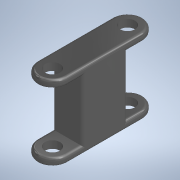
# Autodesk Inventor part: Link2
Saved by Autodesk Inventor 2022 (Build 260153000, 153)
## iProperties
Part Number: Link2
Material: Generic
Document SubType Name: Modeling
Designer: suhas
Appearance: Default
Author: suhas
Autodesk Inventor part; units mm, degrees
ref_plane "YZ Plane" through (0, 0, 0) normal (1, 0, 0) x (0, 1, 0)
ref_plane "XZ Plane" through (0, 0, 0) normal (0, 1, 0) x (-1, 0, 0)
ref_plane "XY Plane" through (0, 0, 0) normal (0, 0, 1) x (1, 0, 0)
sketch "Sketch1" plane through (0, 0, 0) normal (0, 1, 0) x (-1, 0, 0)
  line L0 (10, -25) -> (10, 25)
  line L1 (-10, 25) -> (-10, -25)
  arc A0 (10, 25) -> (-10, 25) centre (0, 25) ccw
  arc A1 (-10, -25) -> (10, -25) centre (0, -25) ccw
  circle A2 centre (0, 25) radius 5
  circle A3 centre (0, -25) radius 5
  point P0 (0, 0)
  constraints: 4 centre point, 4 end point, 4 point on circle, 2 coincident, 1 parallel, 1 tangent
extrude "Extrusion1" add sketch "Sketch1" along normal blind 50
sketch "Sketch2" plane through (-10, 0, -25) normal (-1, 0, 0) x (0, 0, 1)
  line L0 (-10, 0) -> (-10, 50) projected
  line L1 (10, 5) -> (-10, 5)
  line L2 (-10, 5) -> (-10, 45)
  line L3 (-10, 45) -> (10, 45)
  line L4 (10, 45) -> (10, 5)
  line L5 (0, 0) -> (0, 50) projected
  point P0 (25, 0)
  dimension "d6" = 40
  constraints: 8 end point, 2 parallel, 1 horizontal, 1 perpendicular, 1 point on line
  measures "d6" distance of L1.end L2.end
extrude "Extrusion2" cut sketch "Sketch2" against normal up to surface (20 mm away)
mirror "Mirror1" about plane through (0, 0, 0) normal (0, 0, 1) of "Extrusion2"
fillet "Fillet1" radius 2 24 edges at (0, 50, -35) (-10, 50, 0) (0, 50, 35) (10, 50, 0) (0, 45, -35) (-10, 45, -20) (10, 45, -20) (10, 25, -15) (10, 25, 15) (10, 45, 20) (-10, 45, 20) (0, 45, 35) (-10, 25, 15) (-10, 5, 20) (10, 5, 20) (0, 5, 35) (10, 0, 0) (0, 0, -35) (-10, 0, 0) (0, 0, 35) (10, 5, -20) (-10, 5, -20) (0, 5, -35) (-10, 25, -15)
body "Solid1"
